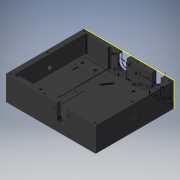
# Autodesk Inventor part: Box_V2
Saved by Autodesk Inventor 2019.4 (Build 234330000, 330)
## iProperties
Created: 2020-06-10
Part Number: Box_V2
Material: Generic
Document SubType Name: Modeling
Designer: ions
Density: 1 g/cm^3
Appearance: Default
Author: ions
Autodesk Inventor part; units mm, degrees
ref_plane "YZ Plane" through (0, 0, 0) normal (1, 0, 0) x (0, 1, 0)
ref_plane "XZ Plane" through (0, 0, 0) normal (0, 1, 0) x (-1, 0, 0)
ref_plane "XY Plane" through (0, 0, 0) normal (0, 0, 1) x (1, 0, 0)
sketch "Sketch1" plane through (0, 0, 0) normal (0, 1, 0) x (-1, 0, 0)
  line L0 (30.5357, 33.6101) -> (-48.4643, 33.6101)
  line L1 (-48.4643, 33.6101) -> (-48.4643, -35.3899)
  line L2 (-48.4643, -35.3899) -> (30.5357, -35.3899)
  line L3 (30.5357, -35.3899) -> (30.5357, 33.6101)
  point P0 (0, 0)
  dimension "d0" = 69
  dimension "d1" = 79
  constraints: 8 end point, 2 parallel, 1 horizontal, 1 perpendicular
  measures "d0" distance between parallel lines of L2 L0
  measures "d1" distance between parallel lines of L1 L3
extrude "Extrusion1" add sketch "Sketch1" along normal blind 21.51
sketch "Sketch2" plane through (0, 21.51, 0) normal (0, 1, 0) x (1, 0, 0)
  line L0 (-6.0357, -29.6101) -> (44.4643, -29.6101)
  line L1 (44.4643, -29.6101) -> (44.4643, 31.3899)
  line L2 (44.4643, 31.3899) -> (-6.0357, 31.3899)
  line L3 (-6.0357, 31.3899) -> (-6.0357, -29.6101)
  line L4 (-30.5357, -33.6101) -> (48.4643, -33.6101) projected
  line L5 (48.4643, -33.6101) -> (48.4643, 35.3899) projected
  line L6 (48.4643, 35.3899) -> (-30.5357, 35.3899) projected
  line L7 (-6.0357, -29.6101) -> (-26.5357, -29.6101)
  line L8 (-26.5357, -29.6101) -> (-26.5357, 31.3899)
  line L9 (-26.5357, 31.3899) -> (-6.0357, 31.3899)
  line L10 (-6.0357, 31.3899) -> (-6.0357, -29.6101)
  line L11 (-30.5357, 35.3899) -> (-30.5357, -33.6101) projected
  point P0 (0, 0)
  dimension "d4" = 4
  dimension "d5" = 4
  dimension "d6" = 4
  dimension "d7" = 50.5
  dimension "d8" = 4
  constraints: 16 end point, 4 parallel, 2 horizontal, 2 perpendicular
  measures "d4" distance between parallel lines of L4 L0
  measures "d5" distance between parallel lines of L5 L1
  measures "d6" distance between parallel lines of L6 L2
  measures "d7" distance between parallel lines of L3 L1
  measures "d8" distance between parallel lines of L11 L8
extrude "Extrusion2" cut sketch "Sketch2" against normal blind 17.51 contours L3 L2 L1 L0
extrude "Extrusion3" cut sketch "Sketch2" against normal blind 15.91 contours L7 L8 L9 L3
sketch "Sketch3" plane through (0, 21.51, 0) normal (0, 1, 0) x (1, 0, 0)
  line L0 (44.4643, -29.6101) -> (-6.0357, -29.6101) projected
  circle A0 centre (42.4643, -29.6101) radius 2
  circle A1 centre (44.4643, 29.3899) radius 2
  circle A2 centre (-4.0357, -29.6101) radius 2
  circle A3 centre (-4.0357, 31.3899) radius 2
  line L1 (-6.0357, -29.6101) -> (-26.5357, -29.6101) projected
  circle A4 centre (-24.5357, -29.6101) radius 2
  circle A5 centre (-24.5357, 31.3899) radius 2
  line L2 (-26.5357, -29.6101) -> (-26.5357, 31.3899) projected
  line L3 (-6.0357, 31.3899) -> (-6.0357, -29.6101) projected
  line L4 (44.4643, 31.3899) -> (44.4643, -29.6101) projected
  line L5 (48.4643, -33.6101) -> (48.4643, 35.3899) projected
  line L6 (48.4643, 35.3899) -> (-30.5357, 35.3899) projected
  point P0 (0, 0)
  dimension "d17" = 4
  dimension "d13" = 4
  dimension "d14" = 2
  dimension "d15" = 4
  dimension "d16" = 2
  dimension "d18" = 4
  dimension "d19" = 2
  dimension "d20" = 4
  dimension "d21" = 2
  dimension "d22" = 4
  dimension "d340" = 4
  dimension "d341" = 4
  constraints: 5 centre point, 3 point on line, 1 horizontal alignment, 2 other
  measures "d13" diameter of A4
  measures "d14" distance of L1.end A4.centre
  measures "d15" diameter of A5
  measures "d16" distance from line of L2 A5.centre
  measures "d18" diameter of A3
  measures "d19" distance from line of L3 A3.centre
  measures "d20" diameter of A0
  measures "d21" distance from line of L4 A0.centre
  measures "d22" diameter of A1
  measures "d340" distance from line of A1.centre L5
  measures "d341" distance edge to line of A1 L6
hole "Hole1" at (42.4643, 21.51, 29.6101) at (-4.0357, 21.51, 29.6101) at (-4.0357, 21.51, -31.3899) direction (0, -1, 0) diameter 4 depth 17.51
hole "Hole2" at (-24.5357, 21.51, 29.6101) at (-24.5357, 21.51, -31.3899) direction (0, -1, 0) diameter 4 depth 15.91
sketch "Sketch4" plane through (0, 4, 0) normal (0, 1, 0) x (1, 0, 0)
  circle A0 centre (39.9643, -24.8601) radius 1.648
  circle A1 centre (21.7143, 26.6399) radius 1.2486
  circle A2 centre (-3.5357, -26.0701) radius 1.0221
  circle A3 centre (-3.5357, 0.8899) radius 1.0142
  line L0 (44.4643, 31.3899) -> (44.4643, -29.6101) projected
  line L1 (44.4643, -29.6101) -> (-6.0357, -29.6101) projected
  line L2 (-6.0357, -29.6101) -> (-6.0357, 31.3899) projected
  point P0 (0, 0)
  point P1 (40.4643, -29.6101)
  point P2 (-2.0357, -29.6101)
  point P3 (44.4643, 30.2913)
  dimension "d38" = 4.5
  dimension "d39" = 4.75
  dimension "d40" = 22.75
  dimension "d41" = 56.25
  dimension "d42" = 2.5
  dimension "d43" = 3.54
  dimension "d44" = 2.5
  dimension "d45" = 26.96
  constraints: 4 centre point
  measures "d38" distance from line of A0.centre L0
  measures "d39" distance from line of A0.centre L1
  measures "d40" distance from line of A1.centre L0
  measures "d41" distance from line of A1.centre L1
  measures "d42" distance from line of A2.centre L2
  measures "d43" distance from line of A2.centre L1
  measures "d44" distance from line of A3.centre L2
  measures "d45" distance of A3.centre A2.centre
hole "Hole3" at (-3.5357, 4, 26.0701) at (-3.5357, 4, -0.8899) direction (0, -1, 0) diameter 1.694 end through all thread size "2-56 UNC" class "2B" standard "ANSI Unified Screw Threads"
hole "Hole4" at (39.9643, 4, 24.8601) at (21.7143, 4, -26.6399) direction (0, -1, 0) diameter 2.642 end through all thread size "6-32 UNC" class "2B" standard "ANSI Unified Screw Threads"
sketch "Sketch5" plane through (0, 5.6, 0) normal (0, 1, 0) x (1, 0, 0)
  circle A0 centre (-24.0357, -26.8601) radius 0.8514
  line L0 (-6.0357, -29.6101) -> (-26.5357, -29.6101) projected
  line L1 (-26.5357, -29.6101) -> (-26.5357, 31.3899) projected
  point P0 (0, 0)
  point P1 (-22.5357, -29.6101)
  dimension "d60" = 2.75
  dimension "d61" = 2.5
  constraints: 1 centre point
  measures "d60" distance from line of A0.centre L0
  measures "d61" distance from line of A0.centre L1
hole "Hole5" at (-24.0357, 5.6, 26.8601) direction (0, -1, 0) diameter 1.694 end through all thread size "2-56 UNC" class "2B" standard "ANSI Unified Screw Threads"
sketch "Sketch6" plane through (-30.5357, 0, 33.6101) normal (0, 0, 1) x (1, 0, 0)
  arc A0 (44.35, 11.23) -> (52.55, 11.23) centre (48.45, 11.23) ccw
  line L0 (79, 0) -> (79, 21.51) projected
  line L1 (0, 21.51) -> (79, 21.51) projected
  line L2 (44.35, 11.23) -> (44.35, 21.51)
  line L3 (52.55, 11.23) -> (52.55, 21.51)
  line L4 (0, 0) -> (79, 0) projected
  point P0 (30.5357, 0)
  dimension "d69" = 30.55
  dimension "d70" = 8.2
  dimension "d364" = 7.13
  constraints: 4 end point, 2 perpendicular, 2 point on circle, 2 point on line, 2 tangent, 1 centre point
  measures "d69" distance from line of A0.centre L0
  measures "d70" diameter of A0
  measures "d364" distance edge to line of A0 L4
extrude "Extrusion4" cut sketch "Sketch6" against normal blind 4
sketch "Sketch7" plane through (48.4643, 0, -35.3899) normal (0, 0, -1) x (-1, 0, 0)
  arc A0 (7.65, 11.23) -> (15.85, 11.23) centre (11.75, 11.23) ccw
  arc A1 (37.5, 13.982) -> (46, 13.982) centre (41.75, 13.982) ccw
  line L0 (0, 0) -> (0, 21.51) projected
  line L1 (0, 21.51) -> (79, 21.51) projected
  line L2 (7.65, 11.23) -> (7.65, 21.51)
  line L3 (50.5, 21.51) -> (4, 21.51) projected
  line L4 (15.85, 11.23) -> (15.85, 21.51)
  line L5 (37.5, 13.982) -> (37.5, 21.51)
  line L6 (46, 13.982) -> (46, 21.51)
  line L7 (79, 21.51) -> (34.65, 21.51) projected
  line L8 (0, 0) -> (79, 0) projected
  point P0 (48.4643, 0)
  point P1 (7.4874, 23.23)
  point P2 (4, 21.51)
  dimension "d74" = 11.75
  dimension "d75" = 41.75
  dimension "d76" = 8.2
  dimension "d78" = 8.5
  dimension "d365" = 7.13
  dimension "d366" = 9.732
  constraints: 8 end point, 4 point on circle, 4 vertical, 3 tangent, 2 centre point, 1 point on line, 5 other
  measures "d74" distance from line of A0.centre L0
  measures "d75" distance from line of A1.centre L0
  measures "d76" diameter of A0
  measures "d78" diameter of A1
  measures "d365" distance edge to line of A0 L8
  measures "d366" distance edge to line of A1 L8
extrude "Extrusion5" cut sketch "Sketch7" against normal blind 4 contours L2 L1 L4 A0
extrude "Extrusion6" cut sketch "Sketch7" against normal blind 4 contours L1 L6 A1 L5
sketch "Sketch8" plane through (0, 4, 0) normal (0, 1, 0) x (1, 0, 0)
  arc A0 (11.1323, 15.8899) -> (12.3393, 18.2805) centre (11.1323, 17.3899) ccw
  arc A1 (1.0926, 18.3449) -> (2.2493, 15.8899) centre (2.2493, 17.3899) ccw
  arc A2 (7.955, 24.7329) -> (5.4773, 24.7383) centre (6.7143, 23.8899) ccw
  line L0 (44.4643, 31.3899) -> (44.4643, -29.6101) projected
  line L1 (44.4643, -29.6101) -> (-6.0357, -29.6101) projected
  line L2 (11.1323, 15.8899) -> (2.2493, 15.8899)
  line L3 (12.3393, 18.2805) -> (7.955, 24.7329)
  line L4 (5.4773, 24.7383) -> (0.9417, 18.1249)
  line L5 (-2.0357, 31.3899) -> (44.4643, 31.3899) projected
  line L6 (33.2143, 31.1999) -> (40.2143, 31.1999)
  line L7 (41.2143, 30.1999) -> (41.2143, 23.1999)
  line L8 (40.2143, 22.1999) -> (33.2143, 22.1999)
  line L9 (32.2143, 23.1999) -> (32.2143, 30.1999)
  arc A3 (33.2143, 31.1999) -> (32.2143, 30.1999) centre (33.2143, 30.1999) ccw
  arc A4 (32.2143, 23.1999) -> (33.2143, 22.1999) centre (33.2143, 23.1999) ccw
  arc A5 (40.2143, 22.1999) -> (41.2143, 23.1999) centre (40.2143, 23.1999) ccw
  arc A6 (41.2143, 30.1999) -> (40.2143, 31.1999) centre (40.2143, 30.1999) ccw
  circle A7 centre (39.9643, -24.8601) radius 1.321 projected
  line L10 (14.4143, -28.4101) -> (21.4143, -28.4101)
  line L11 (22.4143, -27.4101) -> (22.4143, -20.4101)
  line L12 (21.4143, -19.4101) -> (14.4143, -19.4101)
  line L13 (13.4143, -20.4101) -> (13.4143, -27.4101)
  arc A8 (13.4143, -27.4101) -> (14.4143, -28.4101) centre (14.4143, -27.4101) ccw
  arc A9 (14.4143, -19.4101) -> (13.4143, -20.4101) centre (14.4143, -20.4101) ccw
  arc A10 (22.4143, -20.4101) -> (21.4143, -19.4101) centre (21.4143, -20.4101) ccw
  arc A11 (21.4143, -28.4101) -> (22.4143, -27.4101) centre (21.4143, -27.4101) ccw
  point P0 (0, 0)
  point P1 (40.4643, -29.6101)
  point P2 (-2.0357, -29.6101)
  point P3 (44.4643, 30.2913)
  dimension "d104" = 47
  dimension "d105" = 47
  dimension "d106" = 53.5
  dimension "d107" = 33.332
  dimension "d108" = 42.215
  dimension "d109" = 37.75
  dimension "d270" = 3
  dimension "d271" = 3
  dimension "d272" = 3
  dimension "d381" = 1
  dimension "d409" = 47.06
  dimension "d411" = 1.25
  dimension "d412" = 9
  dimension "d413" = 9
  dimension "d414" = 9
  dimension "d415" = 9
  dimension "d416" = 17.55
  dimension "d417" = 3.55
  dimension "d418" = 1
  constraints: 23 point on circle, 22 end point, 19 tangent, 11 centre point, 6 equal radius, 4 parallel, 2 horizontal, 2 perpendicular, 1 point on line
  measures "d104" distance from line of L1 A0.centre
  measures "d105" distance from line of L1 A1.centre
  measures "d106" distance from line of L1 A2.centre
  measures "d107" distance from line of L0 A0.centre
  measures "d108" distance from line of L0 A1.centre
  measures "d109" distance from line of L0 A2.centre
  measures "d270" diameter of A1
  measures "d271" diameter of A2
  measures "d272" diameter of A0
  measures "d381" radius of A3
  measures "d409" distance from line of L8 A7.centre
  measures "d411" distance from line of L7 A7.centre
  measures "d412" distance between parallel lines of L9 L7
  measures "d413" distance between parallel lines of L6 L8
  measures "d414" distance between parallel lines of L11 L13
  measures "d415" distance between parallel lines of L12 L10
  measures "d416" distance from line of L11 A7.centre
  measures "d417" distance from line of L10 A7.centre
  measures "d418" radius of A8
sketch "Sketch9" plane through (0, 4, 0) normal (0, 1, 0) x (1, 0, 0)
  arc A0 (37.1643, -10.0101) -> (39.6643, -10.0101) centre (38.4143, -10.0101) ccw
  arc A1 (39.6643, -6.6101) -> (37.1643, -6.6101) centre (38.4143, -6.6101) ccw
  line L0 (44.4643, -29.6101) -> (-6.0357, -29.6101) projected
  line L1 (44.4643, 31.3899) -> (44.4643, -29.6101) projected
  line L2 (37.1643, -10.0101) -> (37.1643, -6.6101)
  line L3 (39.6643, -10.0101) -> (39.6643, -6.6101)
  line L4 (4.4643, -25.9978) -> (1.8572, -26.0001)
  line L5 (5.5934, -26.4718) -> (-0.1677, -26.4718)
  line L6 (-0.9177, -25.7218) -> (-0.9177, 4.7714)
  line L7 (-0.1677, 5.5214) -> (5.5934, 5.5214)
  line L8 (6.3434, 4.7714) -> (6.3434, -25.7218)
  arc A2 (5.5934, -26.4718) -> (6.3434, -25.7218) centre (5.5934, -25.7218) ccw
  arc A3 (-0.9177, -25.7218) -> (-0.1677, -26.4718) centre (-0.1677, -25.7218) ccw
  arc A4 (-0.1677, 5.5214) -> (-0.9177, 4.7714) centre (-0.1677, 4.7714) ccw
  arc A5 (6.3434, 4.7714) -> (5.5934, 5.5214) centre (5.5934, 4.7714) ccw
  point P0 (0, 0)
  point P1 (40.4643, -29.6101)
  point P2 (-2.0357, -29.6101)
  point P3 (-0.5031, -8.4848)
  point P4 (44.4643, 30.2913)
  dimension "d117" = 19.6
  dimension "d118" = 23
  dimension "d119" = 6.05
  dimension "d120" = 6.05
  dimension "d279" = 2.5
  dimension "d280" = 2.5
  dimension "d293" = 0.75
  constraints: 14 end point, 12 point on circle, 9 tangent, 6 centre point, 3 equal radius, 3 parallel, 1 horizontal, 1 perpendicular
  measures "d117" distance from line of A0.centre L0
  measures "d118" distance from line of L0 A1.centre
  measures "d119" distance from line of A0.centre L1
  measures "d120" distance from line of L1 A1.centre
  measures "d279" diameter of A1
  measures "d280" diameter of A0
  measures "d293" radius of A2
sketch "Sketch10" plane through (0, 5.6, 0) normal (0, 1, 0) x (1, 0, 0)
  circle A0 centre (-11.8257, 15.4999) radius 0.9944
  circle A1 centre (-10.5557, 18.0399) radius 0.8554
  circle A2 centre (-7.0657, 20.4999) radius 0.541
  circle A3 centre (-9.2857, 24.3899) radius 1.3546
  circle A4 centre (-3.5357, -26.0701) radius 0.847 projected
  point P0 (0, 0)
  dimension "d151" = 41.57
  dimension "d152" = 44.11
  dimension "d153" = 46.57
  dimension "d154" = 50.46
  dimension "d155" = 8.29
  dimension "d156" = 3.53
  dimension "d157" = 5.75
  dimension "d158" = 7.02
  constraints: 4 centre point
  measures "d151" vertical distance of A0.centre A4.centre
  measures "d152" vertical distance of A1.centre A4.centre
  measures "d153" vertical distance of A2.centre A4.centre
  measures "d154" vertical distance of A3.centre A4.centre
  measures "d155" horizontal distance of A0.centre A4.centre
  measures "d156" horizontal distance of A2.centre A4.centre
  measures "d157" horizontal distance of A3.centre A4.centre
  measures "d158" horizontal distance of A1.centre A4.centre
hole "Hole9" at (-7.0657, 5.6, -20.4999) direction (0, -1, 0) diameter 1.75 depth 2
pattern_linear "Rectangular Pattern2" count 2 spacing 15.87 along (-1, 0, 0) of "Hole9"
hole "Hole10" at (-9.2857, 5.6, -24.3899) direction (0, -1, 0) diameter 3.75 depth 2
pattern_linear "Rectangular Pattern3" count 2 spacing 11.43 along (-1, 0, 0) of "Hole10"
sketch "Sketch12" plane through (0, 5.6, 0) normal (0, 1, 0) x (1, 0, 0)
  arc A0 (-21.5357, -24.4501) -> (-21.5357, -22.4501) centre (-21.5357, -23.4501) ccw
  arc A1 (-25.2937, -22.4501) -> (-25.2937, -24.4501) centre (-25.2937, -23.4501) ccw
  arc A2 (-23.9356, -3.3982) -> (-21.9383, -3.3381) centre (-22.9357, -3.4101) ccw
  arc A3 (-21.9383, 1.2198) -> (-23.9356, 1.3038) centre (-22.9357, 1.2919) ccw
  arc A4 (-17.9857, 5.8899) -> (-17.9857, 3.8899) centre (-17.9857, 4.8899) ccw
  arc A5 (-9.2857, 3.8899) -> (-9.2857, 5.8899) centre (-9.2857, 4.8899) ccw
  circle A6 centre (-3.5357, -26.0701) radius 0.847 projected
  line L0 (-21.5357, -24.4501) -> (-25.2937, -24.4501)
  line L1 (-21.5357, -22.4501) -> (-25.2937, -22.4501)
  line L2 (-23.9356, -3.3982) -> (-23.9356, 1.3038)
  line L3 (-21.9383, -3.3381) -> (-21.9383, 1.2198)
  line L4 (-17.9857, 3.8899) -> (-9.2857, 3.8899)
  line L5 (-17.9857, 5.8899) -> (-9.2857, 5.8899)
  line L6 (-15.5357, -11.6101) -> (-18.3357, -11.6101)
  line L7 (-19.0857, -10.8601) -> (-19.0857, -2.8601)
  line L8 (-18.3357, -2.1101) -> (-15.5357, -2.1101)
  line L9 (-14.7857, -2.8601) -> (-14.7857, -10.8601)
  arc A7 (-15.5357, -11.6101) -> (-14.7857, -10.8601) centre (-15.5357, -10.8601) ccw
  arc A8 (-19.0857, -10.8601) -> (-18.3357, -11.6101) centre (-18.3357, -10.8601) ccw
  arc A9 (-18.3357, -2.1101) -> (-19.0857, -2.8601) centre (-18.3357, -2.8601) ccw
  arc A10 (-14.7857, -2.8601) -> (-15.5357, -2.1101) centre (-15.5357, -2.8601) ccw
  line L10 (-26.5357, -29.6101) -> (-26.5357, 31.3899) projected
  line L11 (-6.0357, -29.6101) -> (-22.5357, -29.6101) projected
  point P0 (0, 0)
  dimension "d197" = 18
  dimension "d198" = 21.758
  dimension "d199" = 2.62
  dimension "d200" = 2.62
  dimension "d201" = 2
  dimension "d202" = 2
  dimension "d203" = 22.66
  dimension "d204" = 27.362
  dimension "d205" = 19.4
  dimension "d206" = 19.4
  dimension "d207" = 2
  dimension "d208" = 2
  dimension "d209" = 5.75
  dimension "d210" = 14.45
  dimension "d211" = 30.96
  dimension "d212" = 30.96
  dimension "d213" = 2
  dimension "d214" = 2
  dimension "d221" = 0.75
  dimension "d423" = 7.45
  dimension "d424" = 11.75
  dimension "d425" = 18
  dimension "d426" = 27.5
  constraints: 20 end point, 20 point on circle, 12 tangent, 10 centre point, 3 equal radius, 3 parallel, 1 horizontal, 1 perpendicular, 1 vertical
  measures "d197" horizontal distance of A0.centre A6.centre
  measures "d198" horizontal distance of A1.centre A6.centre
  measures "d199" vertical distance of A0.centre A6.centre
  measures "d200" vertical distance of A6.centre A1.centre
  measures "d201" diameter of A1
  measures "d202" diameter of A0
  measures "d203" vertical distance of A2.centre A6.centre
  measures "d204" vertical distance of A3.centre A6.centre
  measures "d205" horizontal distance of A2.centre A6.centre
  measures "d206" horizontal distance of A3.centre A6.centre
  measures "d207" diameter of A3
  measures "d208" diameter of A2
  measures "d209" horizontal distance of A5.centre A6.centre
  measures "d210" horizontal distance of A4.centre A6.centre
  measures "d211" vertical distance of A5.centre A6.centre
  measures "d212" vertical distance of A4.centre A6.centre
  measures "d213" diameter of A4
  measures "d214" diameter of A5
  measures "d221" radius of A7
  measures "d423" distance between parallel lines of L7 L10
  measures "d424" distance between parallel lines of L9 L10
  measures "d425" distance between parallel lines of L6 L11
  measures "d426" distance between parallel lines of L8 L11
extrude "Extrusion9" cut sketch "Sketch12" against normal blind 0.5 contours L0 A1 L1 A0
extrude "Extrusion10" cut sketch "Sketch12" against normal blind 0.5 contours L2 A3 L3 A2
extrude "Extrusion11" cut sketch "Sketch12" against normal blind 0.5 contours L5 A5 L4 A4
extrude "Extrusion13" cut sketch "Sketch12" against normal blind 0.5 contours L6 A8 L7 A9 L8 A10 L9 A7
sketch "Sketch13" plane through (0, 5.6, 0) normal (0, 1, 0) x (1, 0, 0)
  circle A0 centre (-3.5357, -26.0701) radius 0.847 projected
  line L0 (-5.53, -8.7095) -> (-9.782, -8.7095)
  line L1 (-13.4006, -4.0679) -> (-13.4006, 1.6911)
  line L2 (-12.4006, 2.6911) -> (-5.53, 2.6911)
  line L3 (-4.53, 1.6911) -> (-4.53, -7.7095)
  line L4 (-10.5939, -8.2933) -> (-13.2125, -4.6518)
  arc A1 (-10.5939, -8.2933) -> (-9.782, -8.7095) centre (-9.782, -7.7095) ccw
  arc A2 (-13.4006, -4.0679) -> (-13.2125, -4.6518) centre (-12.4006, -4.0679) ccw
  arc A3 (-12.4006, 2.6911) -> (-13.4006, 1.6911) centre (-12.4006, 1.6911) ccw
  arc A4 (-4.53, 1.6911) -> (-5.53, 2.6911) centre (-5.53, 1.6911) ccw
  arc A5 (-5.53, -8.7095) -> (-4.53, -7.7095) centre (-5.53, -7.7095) ccw
  line L5 (-6.0357, -29.6101) -> (-6.0357, 31.3899) projected
  line L6 (-6.0357, -26.4806) -> (-6.656, -26.4806)
  line L7 (-16.6402, -19.3165) -> (-16.6402, -18.9782)
  line L8 (-10.2728, -12.6411) -> (-6.0357, -12.6411)
  line L9 (-6.0357, -12.6411) -> (-6.0357, -26.4806)
  line L10 (-16.3453, -18.2691) -> (-10.9779, -12.932)
  line L11 (-15.6402, -20.3165) -> (-7.656, -20.3165)
  line L12 (-7.656, -20.3165) -> (-7.656, -25.4806)
  arc A6 (-10.2728, -12.6411) -> (-10.9779, -12.932) centre (-10.2728, -13.6411) ccw
  arc A7 (-16.6402, -19.3165) -> (-15.6402, -20.3165) centre (-15.6402, -19.3165) ccw
  arc A8 (-16.3453, -18.2691) -> (-16.6402, -18.9782) centre (-15.6402, -18.9782) ccw
  arc A9 (-7.656, -25.4806) -> (-6.656, -26.4806) centre (-6.656, -25.4806) ccw
  point P0 (0, 0)
  dimension "d427" = 1
  dimension "d428" = 1
  dimension "d429" = 1
  constraints: 24 end point, 18 point on circle, 18 tangent, 9 centre point, 6 equal radius, 4 parallel, 3 horizontal, 3 perpendicular, 1 point on line
  measures "d427" radius of A1
  measures "d428" radius of A6
  measures "d429" radius of A9
extrude "Extrusion14" cut sketch "Sketch13" against normal blind 0.5 contours L5 L6 A9 L12 L11 A7 L7 A8 L10 A6 L8
extrude "Extrusion15" cut sketch "Sketch13" against normal blind 0.5 contours L0 L5 L2 A4 L3 A5 | L0 A1 L4 A2 L1 A3 L2 L5
extrude "Extrusion17" cut sketch "Sketch8" against normal blind 2 contours A8 L13 A9 L12 A10 L11 A11 L10
extrude "Extrusion18" cut sketch "Sketch8" against normal blind 2 contours L2 A1 L4 A2 L3 A0 | A1 L4
extrude "Extrusion19" cut sketch "Sketch8" against normal blind 2 contours L6 A6 L7 A5 L8 A4 L9 A3
extrude "Extrusion20" cut sketch "Sketch9" against normal blind 2 contours L2 A1 L3 A0
sketch "Sketch14" plane through (0, 5.6, 0) normal (0, 1, 0) x (1, 0, 0)
  line L0 (-20.3857, 13.9899) -> (-9.7857, 13.9899)
  line L1 (-9.0357, 14.7399) -> (-9.0357, 19.1399)
  line L2 (-9.7857, 19.8899) -> (-20.3857, 19.8899)
  line L3 (-21.1357, 19.1399) -> (-21.1357, 14.7399)
  arc A0 (-21.1357, 14.7399) -> (-20.3857, 13.9899) centre (-20.3857, 14.7399) ccw
  arc A1 (-20.3857, 19.8899) -> (-21.1357, 19.1399) centre (-20.3857, 19.1399) ccw
  arc A2 (-9.7857, 13.9899) -> (-9.0357, 14.7399) centre (-9.7857, 14.7399) ccw
  arc A3 (-9.0357, 19.1399) -> (-9.7857, 19.8899) centre (-9.7857, 19.1399) ccw
  line L4 (-26.5357, -29.6101) -> (-26.5357, 31.3899) projected
  line L5 (-22.5357, 31.3899) -> (-6.0357, 31.3899) projected
  point P0 (0, 0)
  dimension "d287" = 0.75
  dimension "d419" = 5.4
  dimension "d420" = 17.5
  dimension "d421" = 17.4
  dimension "d422" = 11.5
  constraints: 8 end point, 8 point on circle, 8 tangent, 4 centre point, 3 equal radius, 2 parallel, 1 horizontal, 1 perpendicular
  measures "d287" radius of A0
  measures "d419" distance between parallel lines of L3 L4
  measures "d420" distance between parallel lines of L1 L4
  measures "d421" distance between parallel lines of L5 L0
  measures "d422" distance between parallel lines of L2 L5
extrude "Extrusion22" cut sketch "Sketch14" against normal blind 2
extrude "Extrusion23" cut sketch "Sketch9" against normal blind 1 contours L5 A3 L6 A4 L7 A5 L8 A2
hole "Hole11" at (44.4643, 21.51, -29.3899) direction (0, -1, 0) diameter 4 depth 17.51
sketch "Sketch17" plane through (48.4643, 0, -35.3899) normal (0, 0, -1) x (-1, 0, 0)
  arc A0 (37.5, 13.982) -> (46, 13.982) centre (41.75, 13.982) ccw projected
  circle A1 centre (41.75, 13.982) radius 7.25
  point P0 (48.4643, 0)
  dimension "d309" = 14.5
  constraints: 1 centre point, 1 coincident
  measures "d309" diameter of A1
extrude "Extrusion26" cut sketch "Sketch17" against normal blind 2
sketch "Sketch18" plane through (0, 21.51, 0) normal (0, 1, 0) x (1, 0, 0)
  circle A0 centre (46.4643, -31.6101) radius 1.0225
  line L0 (22.0143, -33.6101) -> (48.4643, -33.6101) projected
  line L1 (48.4643, -33.6101) -> (48.4643, 35.3899) projected
  line L2 (48.4643, 35.3899) -> (40.8143, 35.3899) projected
  circle A1 centre (1.4643, -31.6101) radius 1.1394
  line L3 (-30.5357, -33.6101) -> (13.8143, -33.6101) projected
  circle A2 centre (18.4643, 33.3899) radius 1.0132
  line L4 (10.9643, 31.3899) -> (32.6143, 31.3899) projected
  line L5 (-30.5357, 35.3899) -> (-30.5357, -33.6101) projected
  point P0 (0, 0)
  dimension "d312" = 2
  dimension "d313" = 2
  dimension "d368" = 2
  dimension "d369" = 2
  dimension "d370" = 30
  dimension "d430" = 32
  constraints: 3 centre point
  measures "d312" distance from line of A0.centre L0
  measures "d313" distance from line of A0.centre L1
  measures "d368" distance from line of A1.centre L3
  measures "d369" distance from line of A2.centre L4
  measures "d370" distance from line of A2.centre L1
  measures "d430" distance from line of L5 A1.centre
hole "Hole12" at (46.4643, 21.51, 31.6101) direction (0, -1, 0) diameter 1.694 depth 6.637 thread size "2-56 UNC" class "2B" standard "ANSI Unified Screw Threads"
pattern_linear "Rectangular Pattern4" count 2 spacing 75 along (-1, 0, 0) count 3 spacing 32.5 along (0, 0, -1) of "Hole12"
sketch "Sketch19" plane through (-2.0357, 4, -31.3899) normal (0, 0, 1) x (1, 0, 0)
  circle A0 centre (1.5, 15.01) radius 1.1114
  circle A1 centre (16, 15.01) radius 1.1114
  line L0 (0, 17.51) -> (4.5, 17.51) projected
  line L1 (13, 17.51) -> (34.65, 17.51) projected
  line L2 (4.5, 9.982) -> (4.5, 17.51) projected
  line L3 (13, 17.51) -> (13, 9.982) projected
  point P0 (2.0357, -4)
  dimension "d329" = 2.5
  dimension "d330" = 2.5
  dimension "d331" = 3
  dimension "d332" = 3
  constraints: 2 centre point
  measures "d329" distance from line of A0.centre L0
  measures "d330" distance from line of A1.centre L1
  measures "d331" distance from line of A0.centre L2
  measures "d332" distance from line of A1.centre L3
hole "Hole13" at (-0.5357, 19.01, -31.3899) at (13.9643, 19.01, -31.3899) direction (0, 0, -1) diameter 1.694 end through all thread size "2-56 UNC" class "2B" standard "ANSI Unified Screw Threads"
sketch "Sketch20" plane through (40.4643, 4, 29.6101) normal (0, 0, -1) x (-1, 0, 0)
  circle A0 centre (16.45, 12.51) radius 0.8228
  circle A1 centre (28.65, 12.51) radius 0.9454
  line L0 (0, 17.51) -> (18.45, 17.51) projected
  line L1 (26.65, 17.51) -> (42.5, 17.51) projected
  line L2 (18.45, 7.23) -> (18.45, 17.51) projected
  line L3 (26.65, 17.51) -> (26.65, 7.23) projected
  point P0 (40.4643, -4)
  dimension "d342" = 5
  dimension "d343" = 5
  dimension "d344" = 2
  dimension "d345" = 2
  constraints: 2 centre point
  measures "d342" distance from line of A0.centre L0
  measures "d343" distance from line of A1.centre L1
  measures "d344" distance from line of A0.centre L2
  measures "d345" distance from line of L3 A1.centre
hole "Hole14" at (24.0143, 16.51, 29.6101) at (11.8143, 16.51, 29.6101) direction (0, 0, 1) diameter 1.694 end through all thread size "2-56 UNC" class "2B" standard "ANSI Unified Screw Threads"
sketch "Sketch21" plane through (-2.0357, 4, -31.3899) normal (0, 0, 1) x (1, 0, 0)
  circle A0 centre (32.65, 12.51) radius 0.9005
  circle A1 centre (44.85, 12.51) radius 1.1761
  line L0 (13, 17.51) -> (34.65, 17.51) projected
  line L1 (34.65, 7.23) -> (34.65, 17.51) projected
  line L2 (42.85, 17.51) -> (46.5, 17.51) projected
  line L3 (42.85, 17.51) -> (42.85, 7.23) projected
  point P0 (2.0357, -4)
  dimension "d353" = 5
  dimension "d354" = 2
  dimension "d355" = 5
  dimension "d356" = 2
  constraints: 2 centre point
  measures "d353" distance from line of A0.centre L0
  measures "d354" distance from line of L1 A0.centre
  measures "d355" distance from line of A1.centre L2
  measures "d356" distance from line of A1.centre L3
hole "Hole15" at (30.6143, 16.51, -31.3899) at (42.8143, 16.51, -31.3899) direction (0, 0, -1) diameter 1.694 end through all thread size "2-56 UNC" class "2B" standard "ANSI Unified Screw Threads"
hole "Hole16" at (1.4643, 21.51, 31.6101) at (18.4643, 21.51, -33.3899) direction (0, -1, 0) diameter 1.694 depth 6.637 thread size "2-56 UNC" class "2B" standard "ANSI Unified Screw Threads"
sketch "Sketch22" plane through (48.4643, 0, 33.6101) normal (1, 0, 0) x (0, 0, -1)
  circle A0 centre (34.5, 10.755) radius 2.3753
  line L0 (0, 0) -> (0, 21.51) projected
  line L1 (0, 21.51) -> (69, 21.51) projected
  point P0 (33.6101, 0)
  dimension "d382" = 34.5
  dimension "d383" = 10.755
  constraints: 1 centre point
  measures "d382" distance from line of A0.centre L0
  measures "d383" distance from line of A0.centre L1
hole "Hole17" at (48.4643, 10.755, -0.8899) direction (-1, 0, 0) diameter 3.302 end through all thread size "8-32 UNC" class "2B" standard "ANSI Unified Screw Threads"
sketch "Sketch23" plane through (0, 4, 0) normal (0, 1, 0) x (1, 0, 0)
  circle A0 centre (36.4643, 16.3899) radius 2.1622
  line L0 (44.4643, 27.3899) -> (44.4643, -29.6101) projected
  line L1 (-2.0357, 31.3899) -> (44.4643, 31.3899) projected
  point P0 (0, 0)
  dimension "d391" = 8
  dimension "d392" = 15
  constraints: 1 centre point
  measures "d391" distance from line of A0.centre L0
  measures "d392" distance from line of A0.centre L1
hole "Hole18" at (36.4643, 4, -16.3899) direction (0, -1, 0) diameter 3.302 end through all thread size "8-32 UNC" class "2B" standard "ANSI Unified Screw Threads"
sketch "Sketch24" plane through (0, 5.6, 0) normal (0, 1, 0) x (1, 0, 0)
  circle A0 centre (-18.5357, -14.6101) radius 1.9224
  line L0 (-26.5357, -29.6101) -> (-26.5357, 31.3899) projected
  line L1 (-6.0357, -29.6101) -> (-22.5357, -29.6101) projected
  point P0 (0, 0)
  dimension "d400" = 8
  dimension "d401" = 15
  constraints: 1 centre point
  measures "d400" distance from line of A0.centre L0
  measures "d401" distance from line of A0.centre L1
hole "Hole19" at (-18.5357, 5.6, 14.6101) direction (0, -1, 0) diameter 3.302 end through all thread size "8-32 UNC" class "2B" standard "ANSI Unified Screw Threads"
body "Solid1"
